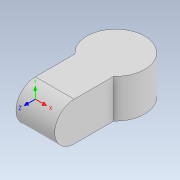
# Autodesk Inventor part: thigh_inventor
Saved by Autodesk Inventor 2020 (Build 240168000, 168)
## iProperties
Created: 2021-01-07
Part Number: thigh_inventor
Material: Generic
Document SubType Name: Modeling
Designer: DELL
Density: 1 g/cm^3
Appearance: Default
Author: DELL
Autodesk Inventor part; units mm, degrees
ref_plane "YZ Plane" through (0, 0, 0) normal (1, 0, 0) x (0, 1, 0)
ref_plane "XZ Plane" through (0, 0, 0) normal (0, 1, 0) x (-1, 0, 0)
ref_plane "XY Plane" through (0, 0, 0) normal (0, 0, 1) x (1, 0, 0)
sketch "Sketch1" plane through (0, 0, 0) normal (0, 1, 0) x (-1, 0, 0)
  line L0 (0, 0) -> (-53, 0)
  line L1 (-53, 0) -> (-53, -83.5)
  line L2 (-53, -83.5) -> (0, -83.5)
  line L3 (0, -83.5) -> (0, 0)
  circle A0 centre (-26.5, -83.5) radius 39.5
  point P0 (-53, -54.2084)
  point P1 (0, -54.2084)
  dimension "d0" = 53
  dimension "d1" = 79
  dimension "d14" = 83.5
  constraints: 8 end point, 2 parallel, 1 centre point, 1 horizontal, 1 midpoint, 1 perpendicular
  measures "d0" distance between parallel lines of L1 L3
  measures "d1" diameter of A0
  measures "d14" distance between parallel lines of L0 L2
extrude "Extrusion1" add sketch "Sketch1" along normal mid plane 53
sketch "Sketch2" plane through (0, 0, 0) normal (1, 0, 0) x (0, 1, 0)
  line L0 (-26.5, 0) -> (26.5, 0) projected
  circle A0 centre (0, 0) radius 26.5
  constraints: 1 midpoint, 3 other
extrude "Extrusion2" add sketch "Sketch2" along normal up to surface (53 mm away) contours A0 L0 picked at (8.0782, 6.219)
body "Solid1"
